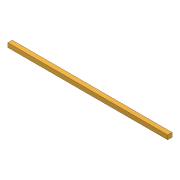
# Autodesk Inventor part: Fret
Saved by Autodesk Inventor 2021 (Build 250183000, 183)
## iProperties
Created: 2021-03-17
Part Number: Fret
Material: Generic
Document SubType Name: Modeling
Designer: Tom
Density: 1 g/cm^3
Appearance: Brass - Satin
Author: Tom
Autodesk Inventor part; units mm, degrees
ref_plane "YZ Plane" through (0, 0, 0) normal (1, 0, 0) x (0, 1, 0)
ref_plane "XZ Plane" through (0, 0, 0) normal (0, 1, 0) x (-1, 0, 0)
ref_plane "XY Plane" through (0, 0, 0) normal (0, 0, 1) x (1, 0, 0)
sketch "Sketch1" plane through (0, 0, 0) normal (1, 0, 0) x (0, 1, 0)
  line L0 (-0.7938, 0.7937) -> (0.7937, 0.7937)
  line L1 (0.7937, 0.7937) -> (0.7938, -0.7937)
  line L2 (0.7938, -0.7937) -> (-0.7937, -0.7937)
  line L3 (-0.7937, -0.7937) -> (-0.7938, 0.7937)
  line L4 (-0.7937, -0.7937) -> (0.7937, 0.7937)
  line L5 (-0.7938, 0.7937) -> (0.7938, -0.7937)
  point P0 (0, 0)
  point P1 (0, 0)
  dimension "d2" = 1.5875
  dimension "d3" = 1.5875
  constraints: 12 end point, 2 parallel, 1 coincident, 1 horizontal, 1 midpoint, 1 perpendicular
  measures "d2" distance of L1.end L2.end
  measures "d3" distance of L0.end L1.end
extrude "Extrusion1" add sketch "Sketch1" against normal blind 58.7375
body "Solid1"
